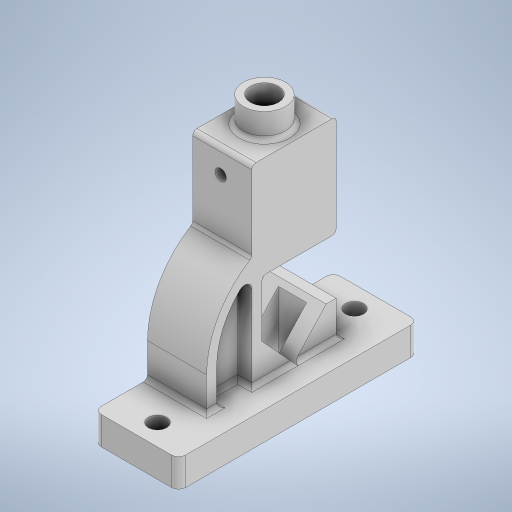
# Autodesk Inventor part: Corps
Saved by Autodesk Inventor 2023.2 (Build 272271030, 271C)
## iProperties
Created: 2023-03-02
Part Number: Corps
Material: Generic
Document SubType Name: Modeling
Designer: Luis Valente
Density: 1 g/cm^3
Appearance: Default
Author: Luis Valente
Autodesk Inventor part; units mm, degrees
ref_plane "XY Plane" through (0, 0, 0) normal (0, 0, 1) x (1, 0, 0)
sketch "Sketch1" plane through (0, 0, 0) normal (0, 1, 0) x (-1, 0, 0)
  line L0 (0, 0) -> (-60, 0)
  line L1 (-60, 0) -> (-60, -170)
  line L2 (-60, -170) -> (0, -170)
  line L3 (0, -170) -> (0, 0)
  dimension "d0" = 60
  dimension "d1" = 170
  constraints: 8 end point, 2 parallel, 1 horizontal, 1 perpendicular
  measures "d0" distance of L2.end L1.end
  measures "d1" distance of L1.end L0.end
extrude "Extrusion1" add sketch "Sketch1" along normal blind 20
fillet "Fillet1" radius 5 4 edges at (60, 10, 0) (0, 10, 0) (60, 10, -170) (0, 10, -170)
sketch "Sketch2" plane through (0, 20, 0) normal (0, 1, 0) x (1, 0, 0)
  line L0 (0, 0) -> (30, 0)
  line L1 (5, 0) -> (55, 0) projected
  line L2 (0, 0) -> (30, 0)
  line L3 (5, 0) -> (55, 0) projected
  line L4 (30, 0) -> (30, 15)
  line L5 (0, 170) -> (30, 170)
  line L6 (55, 170) -> (5, 170) projected
  line L7 (30, 170) -> (30, 155)
  circle A0 centre (30, 155) radius 6.5
  circle A1 centre (30, 15) radius 6.5
  dimension "d5" = 15
  dimension "d7" = 15
  dimension "d9" = 13
  dimension "d10" = 13
  constraints: 10 end point, 2 centre point, 2 coincident, 2 midpoint, 1 collinear, 1 perpendicular, 1 vertical
  measures "d5" distance of L0.end L4.end
  measures "d7" distance of L5.end L7.end
  measures "d9" diameter of A0
  measures "d10" diameter of A1
extrude "Extrusion2" cut sketch "Sketch2" against normal blind 20
sketch "Sketch9" plane through (0, 20, 0) normal (0, 1, 0) x (1, 0, 0)
  line L0 (0, 170) -> (0, 100)
  line L1 (0, 165) -> (0, 5) projected
  line L2 (0, 100) -> (0, 130)
  line L3 (0, 130) -> (42, 130)
  line L4 (42, 130) -> (42, 70)
  line L5 (42, 70) -> (0, 70)
  line L6 (0, 70) -> (0, 130)
  point P0 (0, 0)
  point P1 (0, 70)
  dimension "d55" = 70
  dimension "d56" = 30
  dimension "d57" = 42
  dimension "d58" = 60
  constraints: 12 end point, 2 parallel, 2 point on line, 1 horizontal, 1 perpendicular
  measures "d55" distance of L0.start L0.end
  measures "d56" distance of L0.end L2.end
  measures "d57" distance of L4.end L5.end
  measures "d58" distance of L3.end L4.end
extrude "Extrusion7" add sketch "Sketch9" along normal blind 25
sketch "Sketch10" plane through (42, 20, -70) normal (1, 0, 0) x (0, 0, -1)
  line L0 (60, 25) -> (0, 25) projected
  line L1 (30, 25) -> (30, 0)
  line L2 (-65, 0) -> (95, 0) projected
  line L3 (30, 0) -> (7.0917, 25)
  line L4 (30, 0) -> (63.9085, 0) construction
  line L5 (30, 0) -> (52.9083, 25)
  line L6 (30, 0) -> (63.9085, 0) construction
  point P0 (-70, -20)
  dimension "d61" = 132.5
  dimension "d62" = 47.5
  constraints: 10 end point, 2 equal length, 2 horizontal, 2 point on line, 1 midpoint, 1 vertical
  measures "d61" angle of L4 L3
  measures "d62" angle of L6 L5
extrude "Extrusion8" cut sketch "Sketch10" against normal blind 42
ref_plane "Work Plane2" through (0, 45, 0) normal (0, 1, 0) x (-1, 0, 0)
sketch "Sketch12" plane through (0, 45, 0) normal (0, 1, 0) x (1, 0, 0)
  line L0 (42, 77.0917) -> (0, 77.0917) projected
  line L1 (42, 70) -> (0, 70) projected
  line L2 (0, 77.0917) -> (42, 77.0917)
  line L3 (42, 77.0917) -> (42, 70)
  line L4 (42, 70) -> (0, 70)
  line L5 (0, 70) -> (0, 77.0917)
  point P0 (0, 0)
  constraints: 8 end point, 2 parallel, 1 horizontal, 1 perpendicular
extrude "Extrusion10" add sketch "Sketch12" along normal blind 40
sketch "Sketch13" plane through (0, 85, 0) normal (0, 1, 0) x (1, 0, 0)
  line L0 (42, 130) -> (42, 100) projected
  line L1 (0, 70) -> (42, 70)
  line L2 (42, 70) -> (42, 130)
  line L3 (42, 130) -> (0, 130)
  line L4 (0, 130) -> (0, 70)
  point P0 (0, 0)
  constraints: 8 end point, 2 parallel, 1 horizontal, 1 perpendicular
extrude "Extrusion11" add sketch "Sketch13" along normal blind 72
fillet "Fillet2" radius 3 4 edges at (21, 157, -130) (21, 157, -70) (21, 85, -130) (21, 85, -77.0917)
sketch "Sketch15" plane through (42, 20, -70) normal (1, 0, 0) x (0, 0, -1)
  line L0 (60, 25) -> (60, 65)
  line L1 (30, 0) -> (0, 0) projected
  line L2 (0, 0) -> (0, 60)
  line L3 (0, -20) -> (0, 40)
  line L4 (0, 40) -> (0, 100)
  line L5 (0, 0) -> (0, 134) projected
  line L6 (0, 40) -> (0, 80)
  line L7 (7.0917, 25) -> (7.0917, 62) projected
  line L8 (7.0917, 25) -> (0, 25)
  line L9 (0, 0) -> (-25, 0)
  line L10 (-25, 0) -> (-32.092, 0)
  line L11 (0, 0) -> (-65, 0) projected
  line L12 (0, 0) -> (-25, 0)
  line L13 (0, 80) -> (0, 0)
  line L14 (-32.092, 0) -> (0, 0)
  line L15 (0, 0) -> (0, 80)
  line L16 (0, 80) -> (-32.092, 80)
  line L17 (-32.092, 80) -> (-32.092, 0)
  point P0 (-70, -20)
  dimension "d79" = 40
  dimension "d83" = 60
  dimension "d85" = 40
  dimension "d86" = 25
  dimension "d87" = 7.092
  constraints: 28 end point, 5 point on line, 3 horizontal, 2 parallel, 2 perpendicular, 1 vertical
  measures "d79" distance of L0.start L0.end
  measures "d83" distance of L3.start L3.end
  measures "d85" distance of L3.end L6.end
  measures "d86" distance of L1.end L9.end
  measures "d87" distance of L9.end L10.end
extrude "Extrusion12" add sketch "Sketch15" against normal blind 42
sketch "Sketch11" plane through (0, 45, 0) normal (0, 1, 0) x (-1, 0, 0)
  line L0 (0, -165) -> (0, -5) projected
  line L1 (0, -129.995) -> (0, -119.995)
  line L2 (0, -119.995) -> (0, -108.995)
  line L3 (0, -119.995) -> (-11, -119.995)
  line L4 (-42, -130) -> (-42, -100) projected
  line L5 (-42, -130) -> (-42, -120)
  line L6 (-42, -120) -> (-31, -120)
  line L7 (-11, -119.995) -> (-31, -119.995)
  line L8 (-31, -119.995) -> (-31, -79.995)
  line L9 (-31, -79.995) -> (-11, -79.995)
  line L10 (-11, -79.995) -> (-11, -119.995)
  point P0 (0, 0)
  dimension "d65" = 10
  dimension "d67" = 11
  dimension "d68" = 10
  dimension "d69" = 11
  dimension "d71" = 40
  constraints: 18 end point, 4 point on line, 3 horizontal, 2 parallel, 1 perpendicular
  measures "d65" distance of L1.start L1.end
  measures "d67" distance of L1.end L3.end
  measures "d68" distance of L4.start L5.end
  measures "d69" distance of L5.end L6.end
  measures "d71" distance of L7.end L8.end
extrude "Extrusion9" cut sketch "Sketch11" along normal blind 102 and the other way blind 44
sketch "Sketch16" plane through (42, 85, -80.0917) normal (1, 0, 0) x (0, 0, -1)
  line L0 (-42.1837, -65) -> (-75.0917, -65) projected
  line L1 (-42.1837, -65) -> (-35.0917, -65)
  line L2 (19.9083, -65) -> (-42.1837, -65) projected
  line L3 (-3, -65) -> (-10.092, -65)
  line L4 (-42.1837, 15) -> (-10.0917, 15) projected
  line L5 (-35.0917, -65) -> (-10.0917, -65)
  line L6 (-10.0917, -65) -> (-10.0917, 15)
  line L7 (-10.0917, 15) -> (19.9083, 15)
  line L8 (-35.0917, -40) -> (-35.0917, -65)
  arc A0 (19.9083, 15) -> (-35.0917, -40) centre (19.9083, -40) ccw
  point P0 (-80.0917, -85)
  point P1 (-10.0917, 6.0977)
  dimension "d90" = 7.092
  dimension "d91" = 7.092
  dimension "d96" = 55
  constraints: 12 end point, 3 point on line, 2 parallel, 2 point on circle, 2 tangent, 1 centre point, 1 horizontal, 1 perpendicular
  measures "d90" distance of L0.start L1.end
  measures "d91" distance of L3.start L3.end
  measures "d96" radius of A0
fillet "Fillet4" radius 65 1 edges at (21, 100, -37.908)
extrude "Extrusion13" cut sketch "Sketch16" against normal blind 10 contours L2 L8 A0 L6
fillet "Fillet6" radius 5 1 edges at (37, 91.0977, -70)
ref_plane "Work Plane4" through (21, 0, 0) normal (1, 0, 0) x (0, 1, 0)
mirror "Mirror1" about plane through (21, 0, 0) normal (1, 0, 0) of "Extrusion13"
mirror "Mirror2" about plane through (21, 0, 0) normal (1, 0, 0) of "Fillet6"
sketch "Sketch19" plane through (0, 157, 0) normal (0, 1, 0) x (1, 0, 0)
  line L0 (0, 127) -> (0, 73) projected
  line L1 (0, 77.0917) -> (0, 100) projected
  line L2 (0, 100) -> (21, 100)
  line L3 (11, 100) -> (0, 100) projected
  circle A0 centre (21, 100) radius 15
  point P0 (0, 0)
  dimension "d104" = 21
  dimension "d105" = 30
  constraints: 2 end point, 1 centre point, 1 coincident, 1 collinear
  measures "d104" distance of L1.end L2.end
  measures "d105" diameter of A0
extrude "Extrusion14" add sketch "Sketch19" along normal blind 18
fillet "Fillet7" radius 3 1 edges at (6, 157, -100)
sketch "Sketch20" plane through (21, 175, -100) normal (0, 1, 0) x (1, 0, 0)
  circle A0 centre (0, 0) radius 10
  dimension "d109" = 20
  constraints: 1 centre point
  measures "d109" diameter of A0
extrude "Extrusion15" cut sketch "Sketch20" against normal blind 28
sketch "Sketch21" plane through (42, 88, -130) normal (0, 0, -1) x (-1, 0, 0)
  line L0 (42, 69) -> (42, 66) projected
  line L1 (42, 69) -> (42, 52)
  line L2 (42, 0) -> (42, 66) projected
  line L3 (42, 52) -> (22, 52)
  circle A0 centre (22, 52) radius 4
  point P0 (42, -88)
  dimension "d112" = 17
  dimension "d113" = 20
  dimension "d114" = 8
  constraints: 4 end point, 1 centre point, 1 coincident, 1 horizontal, 1 point on line
  measures "d112" distance of L0.start L1.end
  measures "d113" distance of L1.end L3.end
  measures "d114" diameter of A0
extrude "Extrusion16" cut sketch "Sketch21" against normal blind 60
fillet "Fillet8" radius 3 9 edges at (42, 20, -41.454) (37, 20, -45) (32, 20, -57.5) (37, 20, -70) (42, 20, -85) (42, 20, -115) (21, 20, -130) (21, 20, -37.908) (21, 100, -70)
body "Solid1"
